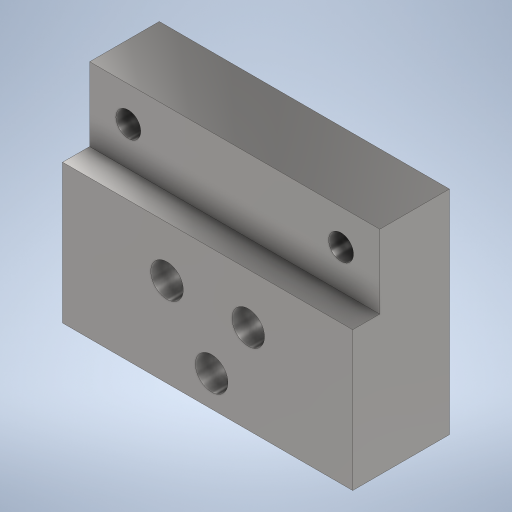
# Autodesk Inventor part: Feste backs
Saved by Autodesk Inventor 2023.2 (Build 272271000, 271)
## iProperties
Created: 2023-02-02
Part Number: Feste backs
Material: Steel, Mild
Document SubType Name: Modeling
Designer: Aditya
Density: 7.85 g/cm^3
Appearance: Semi-Polished
Author: Aditya
Autodesk Inventor part; units mm, degrees
ref_plane "YZ Plane" through (0, 0, 0) normal (1, 0, 0) x (0, 1, 0)
ref_plane "XZ Plane" through (0, 0, 0) normal (0, 1, 0) x (-1, 0, 0)
ref_plane "XY Plane" through (0, 0, 0) normal (0, 0, 1) x (1, 0, 0)
sketch "Sketch1" plane through (0, 0, 0) normal (1, 0, 0) x (0, 1, 0)
  line L0 (0, 0) -> (55, 0)
  line L1 (55, 0) -> (55, 18)
  line L2 (55, 18) -> (36, 18)
  line L3 (36, 18) -> (36, 25)
  line L4 (36, 25) -> (0, 25)
  line L5 (0, 25) -> (0, 0)
  dimension "d0" = 55
  dimension "d1" = 18
  dimension "d2" = 19
  dimension "d3" = 7
  dimension "d4" = 36
  constraints: 12 end point, 4 perpendicular, 1 horizontal
  measures "d0" distance of L0.start L0.end
  measures "d1" distance of L0.end L1.end
  measures "d2" distance of L1.end L2.end
  measures "d3" distance of L2.end L3.end
  measures "d4" distance of L3.end L4.end
extrude "Extrusion1" add sketch "Sketch1" against normal blind 75
sketch "Sketch2" plane through (0, 0, 0) normal (0, 0, -1) x (-1, 0, 0)
  line L0 (0, 0) -> (75, 0) projected
  line L1 (0, 0) -> (0, 55) projected
  line L2 (75, 55) -> (75, 0) projected
  point P0 (27, 23)
  point P1 (48, 23)
  point P2 (36.4618, 8)
  dimension "d7" = 8
  dimension "d15" = 23
  dimension "d16" = 23
  dimension "d26" = 36.4618
  dimension "d27" = 27
  dimension "d28" = 27
  measures "d7" distance from line of L0 point (36.462, 8)
  measures "d15" distance from line of L0 point (48, 23)
  measures "d16" distance from line of L0 point (27, 23)
  measures "d26" distance from line of L1 point (36.462, 8)
  measures "d27" distance from line of L1 point (27, 23)
  measures "d28" distance from line of L2 point (48, 23)
hole "Hole1" at (-36.4618, 8, 0) at (-27, 23, 0) at (-48, 23, 0) direction (0, 0, 1) diameter 8.4 end through all counterbore diameter 15 counterbore depth 10
sketch "Sketch3" plane through (0, 0, 0) normal (0, 0, -1) x (-1, 0, 0)
  line L0 (0, 0) -> (0, 55) projected
  line L1 (75, 55) -> (75, 0) projected
  line L2 (0, 0) -> (75, 0) projected
  point P0 (10, 46)
  point P1 (65, 46)
  dimension "d17" = 10
  dimension "d18" = 10
  dimension "d29" = 46
  dimension "d30" = 46
  measures "d17" distance from line of L0 point (10, 46)
  measures "d18" distance from line of L1 point (65, 46)
  measures "d29" distance from line of L2 point (10, 46)
  measures "d30" distance from line of L2 point (65, 46)
hole "Hole2" at (-10, 46, 0) at (-65, 46, 0) direction (0, 0, 1) diameter 6.4 end through all counterbore diameter 11 counterbore depth 7
body "Solid1"
